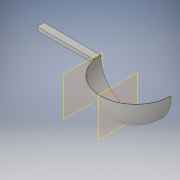
# Autodesk Inventor part: oneHalfSaladBowl
Saved by Autodesk Inventor 2016 SP1 (Build 200210100, 210)
## iProperties
Created: 2016-01-20
Part Number: oneHalfSaladBowl
Material: Generic
Document SubType Name: Modeling
Designer: steele
Density: 1 g/cm^3
Appearance: Default
Author: steele
Autodesk Inventor part; units mm, degrees
ref_plane "XZ Plane" through (0, 0, 0) normal (0, 1, 0) x (-1, 0, 0)
ref_plane "XY Plane" through (0, 0, 0) normal (0, 0, 1) x (1, 0, 0)
sketch "Sketch1" plane through (0, 0, 0) normal (0, 0, 1) x (1, 0, 0)
  arc A0 (0, -127) -> (127, 0) centre (0, 0) ccw
  arc A1 (0, -128.27) -> (128.27, 0) centre (0, 0) ccw
  line L0 (127, 0) -> (128.27, 0)
  line L1 (0, -127) -> (0, -128.27)
  line L2 (0, -185.8027) -> (0, 30.9671) projected
  dimension "d0" = 254
  dimension "d1" = 256.54
  constraints: 4 end point, 4 point on circle, 2 centre point, 2 coincident, 1 horizontal, 1 perpendicular
  measures "d0" diameter of A0
  measures "d1" diameter of A1
revolve "Revolution1" add sketch "Sketch1" angle 180 about axis through (0, -10, 0) along (0, -1, 0)
ref_plane "Work Plane1" through (-128.27, 0, 0) normal (1, 0, 0) x (0, 1, 0)
sketch "Sketch2" plane through (-128.27, 0, 0) normal (1, 0, 0) x (0, 1, 0)
  line L0 (-127, 0) -> (0, 0) projected
  line L1 (0, 0) -> (-12.7, 0)
  line L2 (-12.7, 0) -> (-12.7, 25.4)
  line L3 (-12.7, 25.4) -> (0, 25.4)
  line L4 (0, 25.4) -> (0, 0)
  dimension "d3" = 25.4
  dimension "d4" = 12.7
  constraints: 8 end point, 2 parallel, 1 horizontal, 1 perpendicular
  measures "d3" distance of L1.end L2.end
  measures "d4" distance of L2.end L3.end
extrude "Extrusion1" add sketch "Sketch2" against normal blind 203.2
body "Solid1"
